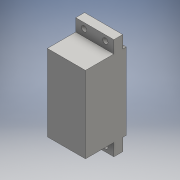
# Autodesk Inventor part: servo
Saved by Autodesk Inventor 2016 (Build 200138000, 138)
## iProperties
Created: 2016-03-04
Part Number: servo
Material: 一般
Document SubType Name: Modeling
Designer: Shun Hasegawa
Density: 1 g/cm^3
Appearance: 既定
Author: Shun Hasegawa
Autodesk Inventor part; units mm, degrees
ref_plane "YZ Plane" through (0, 0, 0) normal (1, 0, 0) x (0, 1, 0)
ref_plane "XZ Plane" through (0, 0, 0) normal (0, 1, 0) x (-1, 0, 0)
ref_plane "XY Plane" through (0, 0, 0) normal (0, 0, 1) x (1, 0, 0)
sketch "スケッチ1" plane through (0, 0, 0) normal (0, 1, 0) x (-1, 0, 0)
  line L0 (10.75, 21.6) -> (-10.75, 21.6)
  line L1 (-10.75, 21.6) -> (-10.75, -21.6)
  line L2 (-10.75, -21.6) -> (10.75, -21.6)
  line L3 (10.75, -21.6) -> (10.75, 21.6)
  line L4 (0, -30.24) -> (0, 30.24) projected
  line L5 (-15.05, 0) -> (15.05, 0) projected
  point P0 (0, 0)
  dimension "d0" = 21.5
  dimension "d1" = 43.2
  constraints: 8 end point, 2 parallel, 1 horizontal, 1 perpendicular, 2 other
  measures "d0" distance of L0.start L0.end
  measures "d1" distance of L2.end L0.start
extrude "押し出し1" add sketch "スケッチ1" along normal blind 16
sketch "スケッチ2" plane through (0, 16, 0) normal (0, 1, 0) x (1, 0, 0)
  line L0 (-10.75, -28.6) -> (10.75, -28.6)
  line L1 (10.75, -28.6) -> (10.75, 28.6)
  line L2 (10.75, 28.6) -> (-10.75, 28.6)
  line L3 (-10.75, 28.6) -> (-10.75, -28.6)
  line L4 (15.155, 0) -> (-15.155, 0) projected
  point P0 (0, 0)
  point P1 (-10.75, -21.6)
  point P2 (10.75, -21.6)
  dimension "d4" = 57.2
  constraints: 8 end point, 2 parallel, 2 point on line, 1 horizontal, 1 perpendicular, 1 other
  measures "d4" distance between parallel lines of L2 L0
extrude "押し出し2" add sketch "スケッチ2" along normal blind 5
sketch "スケッチ3" plane through (0, 21, 0) normal (0, 1, 0) x (1, 0, 0)
  circle A0 centre (-6, -25.6) radius 1.5
  circle A1 centre (6, -25.6) radius 1.5
  circle A2 centre (-6, 25.6) radius 1.5
  circle A3 centre (6, 25.6) radius 1.5
  line L0 (15.05, 0) -> (-15.05, 0) projected
  line L1 (0, 40.04) -> (0, -40.04) projected
  point P0 (0, 0)
  dimension "d9" = 3
  dimension "d10" = 3
  dimension "d11" = 3
  dimension "d12" = 3
  dimension "d13" = 12
  dimension "d14" = 12
  dimension "d15" = 51.2
  dimension "d16" = 51.2
  constraints: 4 centre point, 2 symmetric about line, 1 horizontal alignment, 1 vertical alignment
  measures "d9" diameter of A0
  measures "d10" diameter of A1
  measures "d11" diameter of A2
  measures "d12" diameter of A3
  measures "d13" distance of A1.centre A0.centre
  measures "d14" distance of A3.centre A2.centre
  measures "d15" distance of A2.centre A0.centre
  measures "d16" distance of A3.centre A1.centre
extrude "押し出し3" cut sketch "スケッチ3" against normal up to next
sketch "スケッチ4" plane through (0, 21, 0) normal (0, 1, 0) x (1, 0, 0)
  line L0 (10.75, 21.6) -> (-10.75, 21.6) projected
  line L1 (-10.75, -21.6) -> (10.75, -21.6) projected
  line L2 (-10.75, 28.6) -> (-10.75, -28.6) projected
  line L3 (10.75, -28.6) -> (10.75, 28.6) projected
  point P0 (0, 0)
extrude "押し出し4" add sketch "スケッチ4" along normal blind 2
sketch "スケッチ5" plane through (0, 23, 0) normal (0, 1, 0) x (1, 0, 0)
  circle A0 centre (0, -11.4) radius 3
  circle A1 centre (6, -25.6) radius 1.5 projected
  line L0 (0, 40.04) -> (0, -40.04) projected
  point P0 (0, 0)
  dimension "d21" = 14.2
  dimension "d22" = 6
  constraints: 1 centre point, 1 point on line
  measures "d21" vertical distance of A0.centre A1.centre
  measures "d22" diameter of A0
extrude "押し出し5" add sketch "スケッチ5" along normal blind 3.6 contours A0 L0 | L0 A0
